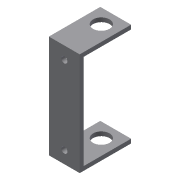
# Autodesk Inventor part: senzor_drzak
Saved by Autodesk Inventor 2015 (Build 190159000, 159)
## iProperties
Created: 2015-03-16
Part Number: senzor_drzak
Material: Generic
Document SubType Name: Modeling
Designer: Turboslimak
Density: 1 g/cm^3
Appearance: Default
Author: Turboslimak
Autodesk Inventor part; units mm, degrees
ref_plane "YZ Plane" through (0, 0, 0) normal (1, 0, 0) x (0, 1, 0)
ref_plane "XZ Plane" through (0, 0, 0) normal (0, 1, 0) x (-1, 0, 0)
ref_plane "XY Plane" through (0, 0, 0) normal (0, 0, 1) x (1, 0, 0)
sketch "Sketch1" plane through (0, 0, 0) normal (0, 1, 0) x (-1, 0, 0)
  line L0 (-7.5, 25) -> (7.5, 25)
  line L1 (7.5, 25) -> (7.5, -25)
  line L2 (7.5, -25) -> (-7.5, -25)
  line L3 (-7.5, -25) -> (-7.5, 25)
  line L4 (-7.5, 25) -> (7.5, -25) construction
  line L5 (7.5, 25) -> (-7.5, -25) construction
  line L6 (0.5, -19) -> (-0.5, -19)
  line L7 (-0.5, 19) -> (0.5, 19)
  circle A0 centre (0, 19) radius 1.5
  circle A1 centre (0, -19) radius 1.5
  line L8 (7.5, -25) -> (-7.5, -25)
  line L9 (-7.5, -25) -> (-7.5, -23)
  line L10 (-7.5, -23) -> (7.5, -23)
  line L11 (7.5, -23) -> (7.5, -25)
  line L12 (7.5, 25) -> (-7.5, 25)
  line L13 (-7.5, 25) -> (-7.5, 23)
  line L14 (-7.5, 23) -> (7.5, 23)
  line L15 (7.5, 23) -> (7.5, 25)
  point P0 (0, 0)
  point P1 (0, 0)
  dimension "d0" = 15
  dimension "d1" = 50
  dimension "d2" = 1
  dimension "d3" = 38
  dimension "d4" = 3
  dimension "d5" = 3
  dimension "d6" = 15
  dimension "d7" = 2
  dimension "d8" = 15
  dimension "d9" = 2
  constraints: 32 end point, 7 parallel, 6 midpoint, 4 horizontal, 3 perpendicular, 2 centre point
  measures "d0" distance of L0.start L0.end
  measures "d1" distance of L0.end L1.end
  measures "d2" distance of L7.start L7.end
  measures "d3" distance of L6.end L7.start
  measures "d4" diameter of A0
  measures "d5" diameter of A1
  measures "d6" distance of L9.end L10.end
  measures "d7" distance of L8.end L9.end
  measures "d8" distance of L14.end L13.end
  measures "d9" distance of L13.end L12.end
extrude "Extrusion1" add sketch "Sketch1" along normal blind 2 contours L14 L1 L10 L3
extrude "Extrusion2" add sketch "Sketch1" along normal blind 25 contours L0 L1 L14 L3 | L10 L1 L2 L3
sketch "Sketch2" plane through (-7.5, 0, 25) normal (0, 0, 1) x (1, 0, 0)
  line L0 (7.5, 0) -> (7.5, 18)
  line L1 (7.5, 0) -> (25.5, 0) construction
  circle A0 centre (7.5, 18) radius 4
  dimension "d14" = 18
  dimension "d15" = 90
  dimension "d16" = 8
  constraints: 4 end point, 1 centre point, 1 coincident, 1 horizontal, 1 perpendicular, 1 vertical
  measures "d14" distance of L0.start L0.end
  measures "d15" angle of L1 L0
  measures "d16" diameter of A0
extrude "Extrusion3" cut sketch "Sketch2" against normal blind 50
body "Solid1"
